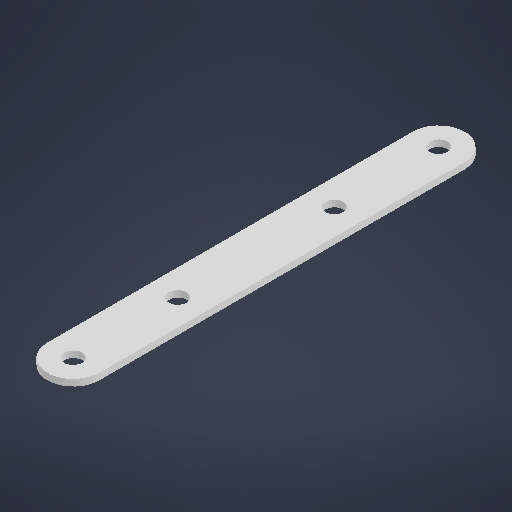
# Autodesk Inventor part: ASD
Saved by Autodesk Inventor 2025.2 (Build 292293000, 293)
## iProperties
Created: 2025-03-26
Part Number: ASD
Material: Generic
Document SubType Name: Modeling
Designer: Jahan
Density: 1 g/cm^3
Appearance: Default
Author: Jahan
Autodesk Inventor part; units mm, degrees
ref_plane "YZ Plane" through (0, 0, 0) normal (1, 0, 0) x (0, 1, 0)
ref_plane "XZ Plane" through (0, 0, 0) normal (0, 1, 0) x (-1, 0, 0)
ref_plane "XY Plane" through (0, 0, 0) normal (0, 0, 1) x (1, 0, 0)
sketch "Sketch1" plane through (0, 0, 0) normal (0, 1, 0) x (-1, 0, 0)
  line L0 (0, 0) -> (0, -25.4)
  line L1 (0, -25.4) -> (0, -63.5)
  line L2 (0, -63.5) -> (0, -88.9)
  line L3 (0, -88.9) -> (0, -114.3)
  circle A0 centre (0, 0) radius 2.1844
  circle A1 centre (0, -25.4) radius 2.1844
  circle A2 centre (0, -63.5) radius 2.1844
  circle A3 centre (0, 0) radius 6.35
  circle A4 centre (0, -88.9) radius 2.1844
  circle A5 centre (0, -88.9) radius 6.35
  line L4 (6.35, -88.9) -> (6.35, 0)
  line L5 (-6.35, -88.9) -> (-6.35, 0)
  dimension "d0" = 25.4
  dimension "d1" = 38.1
  dimension "d2" = 25.4
  dimension "d3" = 25.4
  dimension "d4" = 4.3688
  dimension "d5" = 4.3688
  dimension "d6" = 4.3688
  dimension "d8" = 12.7
  dimension "d12" = 4.3688
  constraints: 12 end point, 6 centre point, 6 coincident, 4 point on circle, 4 tangent, 3 point on line, 3 vertical
  measures "d0" distance of L0.start L0.end
  measures "d1" distance of L0.end L1.end
  measures "d2" distance of L1.end L2.end
  measures "d3" distance of L2.end L3.end
  measures "d4" diameter of A0
  measures "d5" diameter of A1
  measures "d6" diameter of A2
  measures "d8" diameter of A3
  measures "d12" diameter of A4
extrude "Extrusion1" add sketch "Sketch1" along normal blind 1.5875 contours A3 | A3 L4 A5 L2 A2 L1 A1 L0 | L0 A1 L1 A2 L2 A5 L5 A3 | A5 L2 A4 L3 | A5 L3 A4 L2
body "Solid1"
